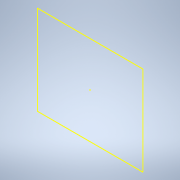
# Autodesk Inventor part: LPS_cap
Saved by Autodesk Inventor 2022 (Build 260153000, 153)
## iProperties
Created: 2024-07-06
Part Number: LPS_cap
Material: Типовые
Document SubType Name: Modeling
Designer: Капустяник Андрей
Density: 1 g/cm^3
Appearance: По умолчанию
Author: Капустяник Андрей
Autodesk Inventor part; units mm, degrees
ref_plane "YZ Plane" through (0, 0, 0) normal (1, 0, 0) x (0, 1, 0)
ref_plane "XZ Plane" through (0, 0, 0) normal (0, 1, 0) x (-1, 0, 0)
ref_plane "XY Plane" through (0, 0, 0) normal (0, 0, 1) x (1, 0, 0)
sketch "Эскиз1" plane through (0, 0, 0) normal (0, 0, 1) x (1, 0, 0)
  line L0 (-68.51, -58) -> (-68.51, 58) projected
  line L1 (-68.51, 58) -> (68.51, 58) projected
  line L2 (68.51, 58) -> (68.51, -58) projected
  line L3 (68.51, -58) -> (-68.51, -58) projected
  point P0 (0, 0)
extrude "Выдавливание1" add sketch "Эскиз1" along normal blind 3
sketch "Эскиз2" plane through (0, 0, 0) normal (0, 0, -1) x (-1, 0, 0)
  line L0 (-65.51, 55) -> (65.51, 55) projected
  line L1 (65.51, 55) -> (65.51, -55) projected
  line L2 (65.51, -55) -> (-65.51, -55) projected
  line L3 (-65.51, -55) -> (-65.51, 55) projected
  line L4 (68.51, -58) -> (68.51, 58) projected
  line L5 (68.51, 58) -> (-68.51, 58) projected
  line L6 (-68.51, 58) -> (-68.51, -58) projected
  line L7 (-68.51, -58) -> (68.51, -58) projected
  point P0 (0, 0)
ref_plane "РабПлоскость1" through (-68.51, -58, -55) normal (0, 0, 1) x (1, 0, 0)
extrude "Выдавливание2" add sketch "Эскиз2" along normal up to surface (55 mm away)
sketch "Эскиз3" plane through (-68.51, 58, 3) normal (0, 1, 0) x (1, 0, 0)
  line L0 (79.02, 58) -> (134.02, 3) projected
  line L1 (3, 3) -> (134.02, 3) projected
  line L2 (0, 58) -> (79.02, 58) projected
  line L3 (79.02, 58) -> (134.02, 3) projected
  line L4 (137.02, 3) -> (134.02, 3) projected
  line L5 (137.02, 3) -> (137.02, 76) projected
  line L6 (0, 76) -> (137.02, 76) projected
  line L7 (0, 58) -> (0, 76) projected
  line L8 (0, 58) -> (137.02, 58) projected
  line L9 (78.5957, 58) -> (133.8079, 2.7879)
  point P0 (68.51, 3)
  point P1 (133.5957, 3)
  dimension "d4" = 0.3
  constraints: 2 end point, 1 parallel, 1 point on line
  measures "d4" distance between parallel lines of L0 L9
extrude "Выдавливание3" cut sketch "Эскиз3" against normal up to surface (116 mm away) contours L8 L5 L4 L0 | L0 L1 L9 L2
